# Autodesk Inventor part: spacer_
Saved by Autodesk Inventor 2016 (Build 200138000, 138)
## iProperties
Created: 2016-07-06
Part Number: spacer_
Material: Generic
Document SubType Name: Modeling
Designer: ajar021
Density: 1 g/cm^3
Appearance: Default
Author: ajar021
Autodesk Inventor part; units mm, degrees
ref_plane "YZ Plane" through (0, 0, 0) normal (1, 0, 0) x (0, 1, 0)
ref_plane "XZ Plane" through (0, 0, 0) normal (0, 1, 0) x (-1, 0, 0)
ref_plane "XY Plane" through (0, 0, 0) normal (0, 0, 1) x (1, 0, 0)
ref_plane "Work Plane1" through (2.9206, -11.5, 0) normal (0, 1, 0) x (1, 0, 0)
sketch "Sketch1" plane through (2.9206, -11.5, 0) normal (0, 1, 0) x (1, 0, 0)
  line L0 (0, 0) -> (30, 0) projected
  line L1 (30, 0) -> (30, 2) projected
  line L2 (20, 2) -> (30, 2) projected
  line L3 (20, 2) -> (20, 4) projected
  line L4 (18, 4) -> (20, 4) projected
  line L5 (18, 2) -> (18, 4) projected
  line L6 (15, 2) -> (18, 2) projected
  line L7 (15, 2) -> (15, 4) projected
  line L8 (13, 4) -> (15, 4) projected
  line L9 (13, 2) -> (13, 4) projected
  line L10 (0, 2) -> (13, 2) projected
  line L11 (0, 0) -> (0, 2) projected
  line L12 (18, 2) -> (18, 0)
  line L13 (18, 2) -> (20, 2)
  line L14 (20, 2) -> (20, 0)
  line L15 (18, 0) -> (20, 0)
  line L16 (18, 0) -> (18, -5)
  line L17 (18, -5) -> (20, -5)
  line L18 (20, -5) -> (20, 0)
  line L19 (18, -5) -> (18, -7)
  line L20 (18, -7) -> (20, -7)
  line L21 (20, -7) -> (20, -5)
  point P0 (-2.9206, 0)
  dimension "d7" = 5
  dimension "d8" = 2
  constraints: 20 end point, 6 perpendicular, 6 point on line, 2 collinear
  measures "d7" distance of L12.end L16.end
  measures "d8" distance of L16.end L19.end
ref_plane "Work Plane2" through (2.9206, -11.5, 0) normal (0, -1, 0) x (1, 0, 0)
extrude "Extrusion3" add sketch "Sketch1" along normal blind 2.5 contours L12 L13 L14 L0 | L0 L18 L17 L16 | L17 L21 L20 L19
sketch "Sketch3" plane through (2.9206, -11.5, 0) normal (0, -1, 0) x (1, 0, 0)
  line L0 (20, 7) -> (20, -2) projected
  line L1 (2, 0) -> (28, 0) projected
  line L2 (20, 0) -> (20, 5)
  line L3 (20, 7) -> (20, -2) projected
  line L4 (20, 5) -> (18, 5)
  line L5 (18, -2) -> (18, 7) projected
  line L6 (18, 5) -> (18, 0)
  line L7 (20, 0) -> (18, 0)
  point P0 (-2.9206, 0)
  dimension "d11" = 5
  constraints: 8 end point, 6 point on line, 1 collinear, 1 perpendicular
  measures "d11" distance of L2.start L2.end
extrude "Extrusion4" add sketch "Sketch3" along normal blind 2.5
body "Solid3"
